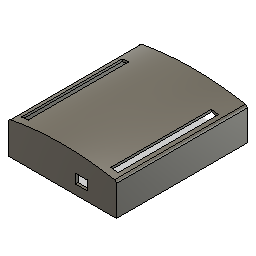
Assembly v19 (Autodesk Fusion 360 archive; units mm, degrees)
design "Cover"
Autodesk Fusion 360 part; units mm, degrees
sketch "Sketch1" plane through (0, 0, 0) normal (0, 0, 1) x (1, 0, 0)
  line L0 (0, 0) -> (58.42, 0)
  line L1 (58.42, 0) -> (58.42, 20.32)
  line L2 (58.42, 20.32) -> (0, 20.32)
  line L3 (0, 20.32) -> (0, 0)
  dimension "d1" = 58.42
  dimension "d2" = 20.32
  constraint horizontal L0
  constraint vertical L1
  constraint horizontal L2
  constraint vertical L3
  constraint coincident L0.start L3.end
  measures "d1" distance of L0.start L0.end
  measures "d2" distance of L0.start L2.end
extrude "Extrude1" add sketch "Sketch1" along normal blind 1.4224
sketch "Sketch2" plane through (0, 0, 0) normal (0, 0, -1) x (-1, 0, 0)
  line L0 (0, 0) -> (0, 20.32)
  line L1 (0, 20.32) -> (-58.42, 20.32)
  line L2 (-58.42, 20.32) -> (-58.42, 0)
  line L3 (-58.42, 0) -> (0, 0)
  circle A0 centre (-29.21, -132.08) radius 152.4
  line L4 (-58.42, 20.32) -> (-29.21, 20.32)
  circle A1 centre (-29.21, -132.08) radius 151.13
  line L5 (-58.42, 0) -> (-57.15, 0)
  line L6 (-57.15, 0) -> (-57.15, 16.4449)
  line L7 (-57.15, 16.4449) -> (-58.42, 16.4449)
  line L8 (-58.42, 16.4449) -> (-58.42, 0)
  line L9 (0, 0) -> (-1.27, 0)
  line L10 (-1.27, 0) -> (-1.27, 16.4449)
  line L11 (-1.27, 16.4449) -> (0, 16.4449)
  line L12 (0, 16.4449) -> (0, 0)
  dimension "d5" = 152.4
  dimension "d6" = 1.27
  dimension "d7" = 1.27
  dimension "d8" = 1.27
  constraint tangent L1 A0
  constraint coincident L1.end L2.start
  constraint midpoint L1 L4.end
  constraint concentric A0 A1
  constraint horizontal L5
  constraint vertical L6
  constraint horizontal L7
  constraint vertical L8
  constraint coincident A1 L6.end
  constraint coincident L2.end L3.start
  constraint horizontal L9
  constraint vertical L10
  constraint horizontal L11
  constraint vertical L12
  constraint coincident A1 L10.end
  constraint coincident L0.start L3.end
  measures "d5" distance of A0.centre L4.end
  measures "d6" distance of A0 A1
  measures "d7" distance of L2.end L5.end
  measures "d8" distance of L0.start L9.end
extrude "Extrude2" add sketch "Sketch2" along normal blind 69.5452 contours L0 L3 A1 L9 L10 L12 | L0 A1 L11 L12 | L0 L2 A0 A1 L7 L11 | L2 L3 A1 L5 L6 L8 | L2 A1 L7 L8
sketch "Sketch4" plane through (0, 20.32, 0) normal (0, 1, 0) x (-1, 0, 0)
  line L0 (-58.42, 0) -> (-29.21, 0)
  line L1 (-29.21, 0) -> (0, 0)
  line L2 (0, 0) -> (0, 1.4224)
  line L3 (0, 1.4224) -> (-58.42, 1.4224)
  line L4 (-58.42, 1.4224) -> (-58.42, 0)
  line L5 (-58.42, 1.4224) -> (-53.467, 1.4224)
  line L6 (-53.467, 1.4224) -> (-53.467, -69.6976)
  line L7 (-53.467, -69.6976) -> (-58.42, -69.6976)
  line L8 (-58.42, -69.6976) -> (-58.42, 1.4224)
  line L9 (0, 1.4224) -> (-4.953, 1.4224)
  line L10 (-4.953, 1.4224) -> (-4.953, -69.6976)
  line L11 (-4.953, -69.6976) -> (0, -69.6976)
  line L12 (0, -69.6976) -> (0, 1.4224)
  line L13 (-53.467, 1.4224) -> (-55.372, 1.4224)
  line L14 (-55.372, 1.4224) -> (-55.372, -69.6976)
  line L15 (-55.372, -69.6976) -> (-53.467, -69.6976)
  line L16 (-53.467, -69.6976) -> (-53.467, 1.4224)
  line L17 (-53.467, 1.4224) -> (-51.562, 1.4224)
  line L18 (-51.562, 1.4224) -> (-51.562, -69.6976)
  line L19 (-51.562, -69.6976) -> (-53.467, -69.6976)
  line L20 (-53.467, -69.6976) -> (-53.467, 1.4224)
  line L21 (-4.953, 1.4224) -> (-3.048, 1.4224)
  line L22 (-3.048, 1.4224) -> (-3.048, -69.6976)
  line L23 (-3.048, -69.6976) -> (-4.953, -69.6976)
  line L24 (-4.953, -69.6976) -> (-4.953, 1.4224)
  line L25 (-4.953, 1.4224) -> (-6.858, 1.4224)
  line L26 (-6.858, 1.4224) -> (-6.858, -69.6976)
  line L27 (-6.858, -69.6976) -> (-4.953, -69.6976)
  line L28 (-4.953, -69.6976) -> (-4.953, 1.4224)
  line L29 (-51.562, -69.6976) -> (-55.372, -69.6976)
  line L30 (-55.372, -69.6976) -> (-55.372, -56.9976)
  line L31 (-55.372, -56.9976) -> (-51.562, -56.9976)
  line L32 (-51.562, -56.9976) -> (-51.562, -69.6976)
  line L33 (-3.048, -69.6976) -> (-6.858, -69.6976)
  line L34 (-6.858, -69.6976) -> (-6.858, -56.9976)
  line L35 (-6.858, -56.9976) -> (-3.048, -56.9976)
  line L36 (-3.048, -56.9976) -> (-3.048, -69.6976)
  line L37 (-3.048, 1.4224) -> (-6.858, 1.4224)
  line L38 (-6.858, 1.4224) -> (-6.858, -2.3876)
  line L39 (-6.858, -2.3876) -> (-3.048, -2.3876)
  line L40 (-3.048, -2.3876) -> (-3.048, 1.4224)
  line L41 (-51.562, 1.4224) -> (-55.372, 1.4224)
  line L42 (-55.372, 1.4224) -> (-55.372, -2.3876)
  line L43 (-55.372, -2.3876) -> (-51.562, -2.3876)
  line L44 (-51.562, -2.3876) -> (-51.562, 1.4224)
  dimension "d26" = 4.953
  dimension "d27" = 71.12
  dimension "d28" = 4.953
  dimension "d29" = 71.12
  dimension "d30" = 1.905
  dimension "d31" = 71.12
  dimension "d32" = 1.905
  dimension "d33" = 71.12
  dimension "d34" = 1.905
  dimension "d35" = 71.12
  dimension "d36" = 1.905
  dimension "d37" = 71.12
  dimension "d38" = 12.7
  dimension "d39" = 12.7
  dimension "d40" = 3.81
  dimension "d41" = 3.81
  constraint horizontal L5
  constraint vertical L6
  constraint horizontal L7
  constraint vertical L8
  constraint coincident L3.end L4.start
  constraint horizontal L9
  constraint vertical L10
  constraint horizontal L11
  constraint vertical L12
  constraint coincident L2.end L3.start
  constraint horizontal L13
  constraint vertical L14
  constraint horizontal L15
  constraint vertical L16
  constraint horizontal L17
  constraint vertical L18
  constraint horizontal L19
  constraint vertical L20
  constraint horizontal L21
  constraint vertical L22
  constraint horizontal L23
  constraint vertical L24
  constraint horizontal L25
  constraint vertical L26
  constraint horizontal L27
  constraint vertical L28
  constraint horizontal L29
  constraint vertical L30
  constraint horizontal L31
  constraint vertical L32
  constraint horizontal L33
  constraint vertical L34
  constraint horizontal L35
  constraint vertical L36
  constraint horizontal L37
  constraint vertical L38
  constraint horizontal L39
  constraint vertical L40
  constraint horizontal L41
  constraint vertical L42
  constraint horizontal L43
  constraint vertical L44
  measures "d26" distance of L3.end L5.end
  measures "d27" distance of L3.end L7.end
  measures "d28" distance of L2.end L9.end
  measures "d29" distance of L2.end L11.end
  measures "d30" distance of L5.end L13.end
  measures "d31" distance of L5.end L6.end
  measures "d32" distance of L5.end L17.end
  measures "d33" distance of L5.end L6.end
  measures "d34" distance of L9.end L21.end
  measures "d35" distance of L9.end L10.end
  measures "d36" distance of L9.end L25.end
  measures "d37" distance of L9.end L10.end
  measures "d38" distance of L18.end L31.end
  measures "d39" distance of L22.end L35.end
  measures "d40" distance of L21.end L39.end
  measures "d41" distance of L17.end L43.end
extrude "Extrude3" cut sketch "Sketch2" against normal up to surface (1.4224 mm away) contours L0 L1 A0 | L1 L2 A0 L4
sketch "Sketch3" plane through (0, 0, 1.4224) normal (0, 0, 1) x (1, 0, 0)
  arc A0 (58.42, 17.4945) -> (0, 17.4945) centre (29.21, -132.08) ccw
  line L0 (0, 17.4945) -> (0, 0)
  line L1 (0, 0) -> (58.42, 0)
  line L2 (58.42, 0) -> (58.42, 17.4945)
  line L3 (36.195, 10.16) -> (42.545, 10.16)
  line L4 (42.545, 10.16) -> (42.545, 5.08)
  line L5 (42.545, 5.08) -> (36.195, 5.08)
  line L6 (36.195, 5.08) -> (36.195, 10.16)
  dimension "d13" = 6.35
  dimension "d14" = 5.08
  dimension "d18" = 5.08
  dimension "d19" = 15.875
  constraint horizontal L3
  constraint vertical L4
  constraint horizontal L5
  constraint vertical L6
  measures "d13" distance of L3.start L3.end
  measures "d14" distance of L3.start L5.end
  measures "d18" distance of L1 L5
  measures "d19" distance of L2 L4
extrude "Extrude4" cut sketch "Sketch3" against normal blind 1.4224 contours L3 L4 L5 L6
fillet "Fillet1" radius 1.27 2 edges at (0, 17.4945, -34.0614) (58.42, 17.4945, -34.0614)
extrude "Extrude5" cut sketch "Sketch4" against normal blind 10.16 contours L6 L14 L16 L20 L31 L43 | L6 L16 L18 L20 L31 L43 | L10 L24 L26 L28 L35 L39 | L10 L22 L24 L28 L35 L39
equation "d26 = 0.05 in + 0.1 in + 0.045 in"
equation "d28 = 0.05 in + 0.1 in + 0.045 in"
